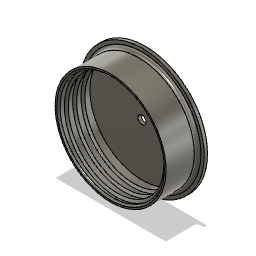
WaterBottleCap_09172021_1340 (Autodesk Fusion 360 design; units mm, degrees)
Autodesk Fusion 360 part; units mm, degrees
note: some values were not read from the file. Set by a fixed rule: which sketch regions a step uses.
sketch "Sketch1" plane through (0, 0, 0) normal (0, 0, 1) x (1, 0, 0)
  circle A0 centre (0, 0) radius 31.5
  dimension "d1" = 63
  constraint coincident A0.centre origin
  measures "d1" diameter of A0
extrude "Extrude1" add sketch "Sketch1" along normal blind 15 makes body 1
shell "Shell1" thickness 2 outward yes removed faces 2 at (10.3827, 15.8486, 15) at (10.3827, 15.8486, 0) on bodies 1
coil "CoilPrimitive1" add diameter 63 section triangle in size 3 on centre turns 3 pitch 5 right hand placed x (1, 0, 0) y (0, 1, 0) z (0, 0, 1) at (0, 0, 0) separate body makes body 2
extrude "Extrude2" add 1 faces at (32.5913, 3.2292, 15) along direction (0, 0, 1) blind 2 on bodies 1 bodies 1 2
extrude "Extrude3" add 1 faces at (-22.9016, 22.4956, 0) along direction (0, 0, -1) blind 2 on bodies 1 bodies 1
sketch "Sketch4" plane through (0, 0, -2) normal (0, 0, -1) x (-1, 0, 0)
  spline S0 degree 3 poles (18.7899, 27.1282) (15.1901, 29.4053) (11.1835, 30.963) (2.8643, 32.4304) (-1.3632, 32.3518) (-8.6803, 30.7552) (-11.7716, 29.5561) (-14.6163, 27.9036) knots 0 0 0 0 1.277846 1.277846 2.535183 2.535183 3.526208 3.526208 3.526208 3.526208
  line L0 (-31.5, 0) -> (-33, 0)
  circle A0 centre (0, 0) radius 37.5
  arc A1 (-31.5, 0) -> (-14.6163, 27.9036) centre (0, 0) ccw
  arc A2 (18.7899, 27.1282) -> (-33, 0) centre (0, 0) ccw
  circle A3 centre (0, 0) radius 33.5
  dimension "d14" = 75
  constraint coincident A0.centre A1.centre
  measures "d14" diameter of A0
extrude "Extrude4" add sketch "Sketch4" along normal blind 2 contours S0 L0 A1 A2 | A0 | A3 bodies 1
sketch "Sketch5" plane through (0, 0, -4) normal (0, 0, -1) x (-1, 0, 0)
  circle A0 centre (0, 0) radius 37.5
  circle A1 centre (0, 0) radius 2.5
  dimension "d17" = 5
  constraint coincident A0.centre A1.centre
  measures "d17" diameter of A1
extrude "Extrude5" cut sketch "Sketch5" against normal blind 11 contours A1 bodies 1
fillet "Fillet3" radius 1 1 edges at (-29.3683, 11.3909, 17) on bodies 1
fillet "Fillet4" radius 2 1 edges at (-31.233, 12.1141, -2) on bodies 1
